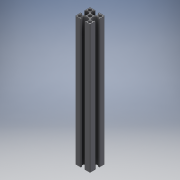
# Autodesk Inventor part: Profile_CPY
Saved by Autodesk Inventor 2016 (Build 200138000, 138)
## iProperties
Created: 2016-12-23
Part Number: Profile_CPY
Material: Generic
Document SubType Name: Modeling
Designer: inorn
Density: 1 g/cm^3
Appearance: Default
Author: inorn
Autodesk Inventor part; units mm, degrees
ref_plane "YZ Plane" through (0, 0, 0) normal (1, 0, 0) x (0, 1, 0)
ref_plane "XZ Plane" through (0, 0, 0) normal (0, 1, 0) x (-1, 0, 0)
ref_plane "XY Plane" through (0, 0, 0) normal (0, 0, 1) x (1, 0, 0)
sketch "Sketch1" plane through (0, 0, 0) normal (0, 0, 1) x (1, 0, 0)
  line L0 (-10, -10) -> (10, 10) construction
  line L1 (10, -10) -> (-10, 10) construction
  arc A0 (-10, -9.5) -> (-9.5, -10) centre (-9.5, -9.5) ccw
  arc A1 (-9.5, 10) -> (-10, 9.5) centre (-9.5, 9.5) ccw
  arc A2 (10, 9.5) -> (9.5, 10) centre (9.5, 9.5) ccw
  arc A3 (9.5, -10) -> (10, -9.5) centre (9.5, -9.5) ccw
  line L2 (7, -7) -> (-7, -7) construction
  line L3 (-7, -7) -> (-7, 7) construction
  line L4 (-7, 7) -> (7, 7) construction
  line L5 (7, 7) -> (7, -7) construction
  line L6 (7, -7) -> (-7, 7) construction
  line L7 (-7, -7) -> (7, 7) construction
  circle A4 centre (-7, -7) radius 2
  circle A5 centre (-7, 7) radius 2
  circle A6 centre (7, 7) radius 2
  circle A7 centre (7, -7) radius 2
  circle A8 centre (0, 0) radius 2.15
  line L8 (-8.5, 4.15) -> (-5.1906, 4.15)
  arc A9 (-5.1906, -4.15) -> (-5.1906, 4.15) centre (-8.8, 0) ccw
  line L9 (-5.1906, -4.15) -> (-8.5, -4.15)
  line L10 (-8.5, -4.15) -> (-8.5, -2.7559)
  line L11 (-8.5, 2.5441) -> (-8.5, 4.15)
  line L12 (-5.1906, -4.15) -> (-5.1906, 4.15) construction
  line L13 (-8.5, -2.7559) -> (-10, -2.7559)
  line L14 (-8.5, 2.5441) -> (-10, 2.5441)
  line L15 (-10, 9.5) -> (-10, 2.5441)
  line L16 (-10, -2.7559) -> (-10, -9.5)
  line L17 (4.15, -8.5) -> (2.7559, -8.5)
  line L18 (2.7559, -8.5) -> (2.7559, -10)
  line L19 (4.15, -5.1906) -> (-4.15, -5.1906) construction
  arc A10 (4.15, -5.1906) -> (-4.15, -5.1906) centre (0, -8.8) ccw
  line L20 (7, -7) -> (-7, 7) construction
  line L21 (10, -10) -> (-10, 10) construction
  line L22 (-4.15, -8.5) -> (-4.15, -5.1906)
  line L23 (4.15, -5.1906) -> (4.15, -8.5)
  line L24 (-2.5441, -8.5) -> (-2.5441, -10)
  line L25 (-2.5441, -8.5) -> (-4.15, -8.5)
  line L26 (8.5, 4.15) -> (8.5, 2.7559)
  line L27 (8.5, 2.7559) -> (10, 2.7559)
  line L28 (5.1906, 4.15) -> (5.1906, -4.15) construction
  arc A11 (5.1906, 4.15) -> (5.1906, -4.15) centre (8.8, 0) ccw
  line L29 (7, 7) -> (-7, -7) construction
  line L30 (10, 10) -> (-10, -10) construction
  line L31 (8.5, -4.15) -> (5.1906, -4.15)
  line L32 (5.1906, 4.15) -> (8.5, 4.15)
  line L33 (8.5, -2.5441) -> (10, -2.5441)
  line L34 (8.5, -2.5441) -> (8.5, -4.15)
  line L35 (-4.15, 8.5) -> (-2.7559, 8.5)
  line L36 (-2.7559, 8.5) -> (-2.7559, 10)
  line L37 (-4.15, 5.1906) -> (4.15, 5.1906) construction
  arc A12 (-4.15, 5.1906) -> (4.15, 5.1906) centre (0, 8.8) ccw
  line L38 (-7, 7) -> (7, -7) construction
  line L39 (-10, 10) -> (10, -10) construction
  line L40 (4.15, 8.5) -> (4.15, 5.1906)
  line L41 (-4.15, 5.1906) -> (-4.15, 8.5)
  line L42 (2.5441, 8.5) -> (2.5441, 10)
  line L43 (2.5441, 8.5) -> (4.15, 8.5)
  line L44 (-9.5, -10) -> (-2.5441, -10)
  line L45 (2.7559, -10) -> (9.5, -10)
  line L46 (9.5, 10) -> (2.5441, 10)
  line L47 (-2.7559, 10) -> (-9.5, 10)
  line L48 (10, -9.5) -> (10, -2.5441)
  line L49 (10, 2.7559) -> (10, 9.5)
  point P0 (-10, 0)
  point P1 (-5.8595, 0)
  point P2 (-5.1906, 0)
  point P3 (-10, 0)
  point P4 (0, -5.8595)
  point P5 (0, -5.1906)
  point P6 (5.8595, 0)
  point P7 (5.1906, 0)
  point P8 (0, 5.8595)
  point P9 (0, 5.1906)
  dimension "d0" = 20
  dimension "d1" = 20
  dimension "d2" = 0.5
  dimension "d3" = 14
  dimension "d4" = 14
  dimension "d5" = 4
  dimension "d6" = 4.3
  dimension "d13" = 5.5
  dimension "d14" = 8.3
  dimension "d16" = 5.3
  dimension "d17" = 6.7
  dimension "d18" = 1.5
  dimension "d21" = 360
  constraints: 100 end point, 16 point on circle, 16 tangent, 13 centre point, 12 parallel, 10 perpendicular, 6 coincident, 6 equal radius, 5 midpoint, 4 horizontal, 1 collinear, 1 point on line, 1 vertical, 102 other
  measures "d0" distance of L1.end L0.end
  measures "d1" distance of L0.end L1.start
  measures "d2" radius of A0
  measures "d3" distance of L3.end L4.end
  measures "d4" distance of L2.end L3.end
  measures "d5" diameter of A4
  measures "d6" diameter of A8
  measures "d13" radius of A9
  measures "d14" distance between parallel lines of L8 L9
  measures "d16" distance between parallel lines of L14 L13
  measures "d18" distance of L11.start L14.end
extrude "Extrusion1" add sketch "Sketch1" along normal blind 176
body "Solid1"
